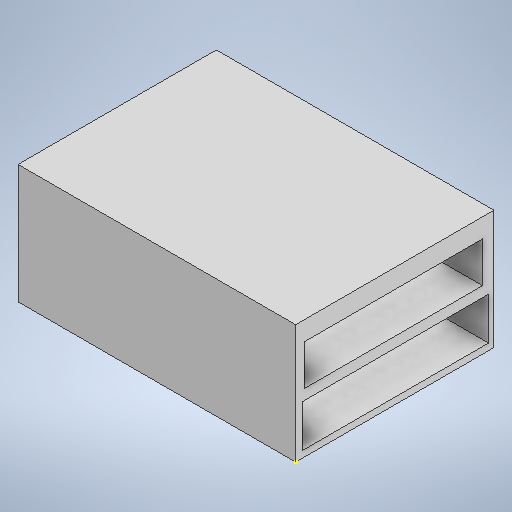
# Autodesk Inventor part: hddcase
Saved by Autodesk Inventor 2025.1 (Build 291241000, 241)
## iProperties
Created: 2024-10-03
Part Number: hddcase
Material: Generic
Document SubType Name: Modeling
Designer: tidal
Density: 1 g/cm^3
Appearance: Default
Author: tidal
Autodesk Inventor part; units mm, degrees
ref_plane "YZ Plane" through (0, 0, 0) normal (1, 0, 0) x (0, 1, 0)
ref_plane "XZ Plane" through (0, 0, 0) normal (0, 1, 0) x (-1, 0, 0)
ref_plane "XY Plane" through (0, 0, 0) normal (0, 0, 1) x (1, 0, 0)
sketch "Sketch1" plane through (0, 0, 0) normal (0, 1, 0) x (-1, 0, 0)
  point P0 (0, 0)
sketch "Sketch2" plane through (0, 0, 0) normal (0, 1, 0) x (-1, 0, 0)
  point P0 (0, 0)
sketch "Sketch3" plane through (0, 0, 0) normal (0, 1, 0) x (-1, 0, 0)
  line L0 (0, 0) -> (140, 0)
  line L1 (140, 0) -> (140, -100)
  line L2 (140, -100) -> (0, -100)
  line L3 (0, -100) -> (0, 0)
  dimension "d0" = 140
  dimension "d1" = 100
  constraints: 8 end point, 2 parallel, 1 horizontal, 1 perpendicular
  measures "d0" distance of L1.end L2.end
  measures "d1" distance of L0.end L1.end
extrude "Extrusion1" add sketch "Sketch3" along normal blind 60
sketch "Sketch4" plane through (0, 0, 0) normal (1, 0, 0) x (0, 0, -1)
  line L0 (3.2517, 3.335) -> (97.2996, 3.335)
  line L1 (97.2996, 3.335) -> (97.2996, 24.6792)
  line L2 (97.2996, 24.6792) -> (3.2517, 24.6792)
  line L3 (3.2517, 24.6792) -> (3.2517, 3.335)
  point P0 (0, 0)
  constraints: 8 end point, 2 parallel, 1 horizontal, 1 perpendicular
extrude "Extrusion2" cut sketch "Sketch4" against normal blind 136.85
sketch "Sketch5" plane through (0, 0, 0) normal (1, 0, 0) x (0, 0, -1)
  line L0 (4.2738, 29.9179) -> (94.2738, 29.9179)
  line L1 (94.2738, 29.9179) -> (94.2738, 50.3488)
  line L2 (94.2738, 50.3488) -> (4.2738, 50.3488)
  line L3 (4.2738, 50.3488) -> (4.2738, 29.9179)
  point P0 (0, 0)
  point P1 (94.2738, 40.1334)
  point P2 (4.2738, 40.1334)
  dimension "d8" = 20.4309
  dimension "d9" = 90
  constraints: 8 end point, 2 midpoint, 2 parallel, 1 horizontal, 1 perpendicular
  measures "d8" distance of L0.end L1.end
  measures "d9" distance of point (94.274, 40.133) point (4.274, 40.133)
extrude "Extrusion3" cut sketch "Sketch5" against normal blind 136.85
body "Solid1"
